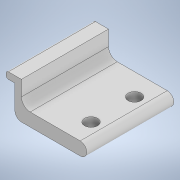
# Autodesk Inventor part: Cable_Guide_Support
Saved by Autodesk Inventor 2021 (Build 250183000, 183)
## iProperties
Created: 2022-01-07
Part Number: Cable_Guide_Support
Material: Generic
Document SubType Name: Modeling
Designer: Jorian Brusind
Density: 1 g/cm^3
Appearance: Default
Author: Jorian Brusind
Autodesk Inventor part; units mm, degrees
ref_plane "YZ Plane" through (0, 0, 0) normal (1, 0, 0) x (0, 1, 0)
ref_plane "XZ Plane" through (0, 0, 0) normal (0, 1, 0) x (-1, 0, 0)
ref_plane "XY Plane" through (0, 0, 0) normal (0, 0, 1) x (1, 0, 0)
sketch "Sketch1" plane through (0, 0, 0) normal (0, 1, 0) x (-1, 0, 0)
  line L0 (0, 0) -> (33, 0)
  line L1 (33, 0) -> (33, -40)
  line L2 (33, -40) -> (0, -40)
  line L3 (0, -40) -> (0, 0)
  dimension "d0" = 33
  dimension "d1" = 40
  constraints: 8 end point, 2 parallel, 1 horizontal, 1 perpendicular
  measures "d0" distance of L1.end L2.end
  measures "d1" distance of L0.end L1.end
extrude "Extrusion1" add sketch "Sketch1" along normal blind 6
sketch "Sketch2" plane through (0, 6, 0) normal (0, 1, 0) x (1, 0, 0)
  line L0 (-33, 0) -> (0, 0) projected
  line L1 (0, 40) -> (-33, 40) projected
  line L2 (-33, 0) -> (-30, 0)
  line L3 (-30, 0) -> (-30, 40)
  line L4 (-30, 40) -> (-33, 40)
  line L5 (-33, 40) -> (-33, 0)
  dimension "d4" = 3
  constraints: 8 end point, 2 parallel, 1 horizontal, 1 perpendicular, 1 point on line
  measures "d4" distance of L4.end L3.end
extrude "Extrusion2" add sketch "Sketch2" along normal blind 11
sketch "Sketch3" plane through (-33, 0, -40) normal (-1, 0, 0) x (0, 0, 1)
  line L0 (0, 17) -> (40, 17) projected
  line L1 (40, 17) -> (0, 17)
  line L2 (0, 17) -> (0, 14)
  line L3 (0, 14) -> (40, 14)
  line L4 (40, 14) -> (40, 17)
  point P0 (40, 0)
  dimension "d7" = 40
  dimension "d8" = 3
  constraints: 8 end point, 2 parallel, 1 horizontal, 1 perpendicular
  measures "d7" distance of L3.end L2.end
  measures "d8" distance of L2.end L1.end
extrude "Extrusion3" add sketch "Sketch3" along normal blind 4
fillet "Fillet1" radius 1 2 edges at (-37, 17, -20) (-37, 14, -20)
fillet "Fillet2" radius 4 1 edges at (-30, 6, -20)
fillet "Fillet3" radius 3 2 edges at (0, 6, -20) (0, 0, -20)
fillet "Fillet4" radius 3 1 edges at (-33, 0, -20)
sketch "Sketch4" plane through (0, 6, 0) normal (0, 1, 0) x (1, 0, 0)
  line L0 (-8, 0) -> (-8, 10)
  line L1 (-3, 40) -> (-30, 40) projected
  circle A0 centre (-8, 10) radius 3
  line L2 (-8, 40) -> (-8, 30)
  line L3 (-8, 40) -> (2, 40) construction
  circle A1 centre (-8, 30) radius 3
  point P0 (0, 0)
  dimension "d15" = 10
  dimension "d16" = 6
  dimension "d17" = 10
  dimension "d18" = 90
  dimension "d19" = 5
  dimension "d20" = 6
  dimension "d23" = 5
  constraints: 6 end point, 2 centre point, 2 coincident, 2 perpendicular, 1 horizontal, 1 point on line, 1 vertical
  measures "d15" distance of L0.start L0.end
  measures "d16" diameter of A0
  measures "d17" distance of L2.start L2.end
  measures "d18" angle of L2 L3
  measures "d19" distance from line of L1.start L2
  measures "d20" diameter of A1
  measures "d23" distance from line of L1.start L0
extrude "Extrusion4" cut sketch "Sketch4" against normal through all
body "Solid1"
